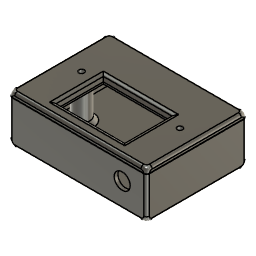
Case (Autodesk Fusion 360 design; units mm, degrees)
part number: 2026-04-11-18-54-48-113
Autodesk Fusion 360 part; units mm, degrees
sketch "Sketch1" plane through (0, 0, 0) normal (0, 0, 1) x (1, 0, 0)
  line L0 (36, -17) -> (-34, -17)
  line L1 (-34, -17) -> (-34, 33)
  line L2 (-34, 33) -> (36, 33)
  line L3 (36, 33) -> (36, -17)
  line L4 (-36, 35) -> (38, 35)
  line L5 (38, 35) -> (38, -19)
  line L6 (38, -19) -> (-36, -19)
  line L7 (-36, -19) -> (-36, 35)
  dimension "d1" = -2
  constraint horizontal L0
  constraint vertical L1
  constraint horizontal L2
  constraint vertical L3
extrude "Extrude1" add sketch "Sketch1" along normal blind 3 contours L0 L1 L2 L3 makes body 1
extrude "Extrude2" add sketch "Sketch1" along normal blind 23 bodies 1
sketch "Sketch2" plane through (-36, 0, 0) normal (-1, 0, 0) x (0, -1, 0)
  line L0 (-35, 0) -> (19, 0)
  line L1 (19, 0) -> (19, 23)
  line L2 (19, 23) -> (-35, 23)
  line L3 (-35, 23) -> (-35, 0)
  line L4 (3.8405, 14.1947) -> (10.2824, 14.1947)
  spline S0 degree 5 poles (10.2824, 14.1947) (10.1277, 14.2067) (9.8414, 14.2278) (9.4814, 14.251) (9.1402, 14.265) (8.9381, 14.255) (8.9359, 14.2207) (9.0834, 14.1681) (9.2938, 14.108) (9.4323, 14.0572) (9.5119, 14.0042) (9.5822, 13.9341) (9.7032, 13.8331) (9.8326, 13.7189) (9.9316, 13.5975) (9.9981, 13.4573) (10.039, 13.2845) (10.0688, 13.0683) (10.0947, 12.8128) (10.114, 12.5387) (10.1198, 12.2727) (10.105, 12.0401) (10.0669, 11.8551) (10.0114, 11.7144) (9.9593, 11.5833) (9.8882, 11.451) (9.7741, 11.3164) (9.6097, 11.1874) (9.4444, 11.0743) (9.3869, 10.985) (9.4842, 10.9238) (9.7088, 10.8991) (9.9628, 10.8944) (10.1702, 10.8974) (10.2835, 10.9005) knots 0 0 0 0 0 0 0.033333 0.066667 0.1 0.133333 0.166667 0.2 0.233333 0.266667 0.3 0.333333 0.366667 0.4 0.433333 0.466667 0.5 0.533333 0.566667 0.6 0.633333 0.666667 0.7 0.733333 0.766667 0.8 0.833333 0.866667 0.9 0.933333 0.966667 1 1 1 1 1 1
  line L5 (10.1343, 12.0688) -> (9.9468, 11.5206)
  line L6 (9.8271, 11.3559) -> (9.3119, 10.9656)
  line L7 (8.9303, 14.2181) -> (9.4188, 14.0666)
  line L8 (9.3851, 14.1073) -> (9.9709, 13.5998)
  line L9 (10.2835, 10.9005) -> (3.8405, 10.9005)
  spline S1 degree 5 poles (10.2824, 14.1947) (10.3107, 14.1924) (10.3649, 14.188) (10.4382, 14.1815) (10.5201, 14.1733) (10.6001, 14.1622) (10.6656, 14.1474) (10.7413, 14.1203) (10.8479, 14.0727) (10.9748, 14.0042) (11.1054, 13.918) (11.221, 13.8196) (11.3211, 13.7164) (11.406, 13.6037) (11.4757, 13.4696) (11.5302, 13.3021) (11.5698, 13.0938) (11.5955, 12.8489) (11.6087, 12.586) (11.6103, 12.3286) (11.6008, 12.1001) (11.5781, 11.9132) (11.5392, 11.7701) (11.4743, 11.6379) (11.3832, 11.4983) (11.2768, 11.3602) (11.1656, 11.2375) (11.0577, 11.1449) (10.9445, 11.0767) (10.8149, 11.0216) (10.6641, 10.9753) (10.5242, 10.9428) (10.4081, 10.9208) (10.3258, 10.9071) (10.2835, 10.9005) knots 0 0 0 0 0 0 0.033333 0.066667 0.1 0.133333 0.166667 0.2 0.233333 0.266667 0.3 0.333333 0.366667 0.4 0.433333 0.466667 0.5 0.533333 0.566667 0.6 0.633333 0.666667 0.7 0.733333 0.766667 0.8 0.833333 0.866667 0.9 0.933333 0.966667 1 1 1 1 1 1
  line L10 (10.4303, 14.2181) -> (10.9188, 14.0666)
  line L11 (10.8851, 14.1073) -> (11.4709, 13.5998)
  line L12 (11.6343, 12.0688) -> (11.4468, 11.5206)
  line L13 (11.3271, 11.3559) -> (10.8119, 10.9656)
  spline S2 degree 5 poles (3.8405, 14.1947) (3.827, 14.1957) (3.7987, 14.1969) (3.7524, 14.1966) (3.6832, 14.1918) (3.585, 14.1778) (3.4774, 14.1546) (3.3667, 14.1181) (3.259, 14.0663) (3.156, 14.0025) (3.0577, 13.9308) (2.9632, 13.854) (2.8723, 13.77) (2.7861, 13.6719) (2.7062, 13.5512) (2.6353, 13.4001) (2.576, 13.2145) (2.5314, 12.9968) (2.5045, 12.7554) (2.4976, 12.5021) (2.5125, 12.2505) (2.5494, 12.0136) (2.6073, 11.8019) (2.683, 11.6212) (2.7715, 11.4716) (2.8677, 11.3495) (2.9685, 11.2496) (3.0732, 11.1659) (3.1882, 11.0945) (3.3197, 11.0332) (3.4705, 10.9806) (3.6079, 10.9447) (3.7205, 10.9213) (3.7998, 10.9072) (3.8405, 10.9005) knots 0 0 0 0 0 0 0.033333 0.066667 0.1 0.133333 0.166667 0.2 0.233333 0.266667 0.3 0.333333 0.366667 0.4 0.433333 0.466667 0.5 0.533333 0.566667 0.6 0.633333 0.666667 0.7 0.733333 0.766667 0.8 0.833333 0.866667 0.9 0.933333 0.966667 1 1 1 1 1 1
  line L14 (3.8606, 14.2596) -> (3.0828, 14.0401)
  line L15 (2.8075, 11.3652) -> (3.311, 10.9966)
  point P0 (9.1746, 14.1424)
  point P1 (9.678, 13.8535)
  point P2 (10.0558, 13.1512)
  point P3 (10.0405, 11.7947)
  point P4 (9.5695, 11.1608)
  point P5 (11.5558, 13.1512)
  point P6 (11.178, 13.8535)
  point P7 (11.5405, 11.7947)
  point P8 (11.0695, 11.1608)
  point P9 (10.6746, 14.1424)
  point P10 (3.4717, 14.1499)
  point P11 (3.011, 13.8917)
  point P12 (2.6182, 13.3365)
  point P13 (2.5919, 11.872)
  point P14 (3.0592, 11.1809)
  constraint horizontal L4
  constraint midpoint P3 L5
  constraint midpoint P4 L6
  constraint midpoint P0 L7
  constraint midpoint P1 L8
  constraint parallel L4 L9
  constraint midpoint P7 L12
  constraint midpoint P8 L13
  constraint midpoint P9 L10
  constraint midpoint P6 L11
  constraint midpoint P10 L14
  constraint midpoint P14 L15
extrude "Extrude3" cut sketch "Sketch2" against normal blind 2 contours L4 S0 L7 L9 S2 bodies 1
sketch "Sketch3" plane through (0, -19, 0) normal (0, -1, 0) x (1, 0, 0)
  line L0 (-36, 0) -> (38, 0)
  line L1 (38, 0) -> (38, 23)
  line L2 (38, 23) -> (-36, 23)
  line L3 (-36, 23) -> (-36, 0)
  circle A0 centre (24.8738, 13.5782) radius 4.325
extrude "Extrude4" cut sketch "Sketch3" against normal blind 2 contours A0 bodies 1
sketch "Sketch4" plane through (0, 0, 23) normal (0, 0, 1) x (-1, 0, 0)
  line L0 (34, -33) -> (-36, -33)
  line L1 (-36, -33) -> (-36, 17)
  line L2 (-36, 17) -> (34, 17)
  line L3 (34, 17) -> (34, -33)
  line L4 (36, 19) -> (-38, 19)
  line L5 (-38, 19) -> (-38, -35)
  line L6 (-38, -35) -> (36, -35)
  line L7 (36, -35) -> (36, 19)
  line L8 (-38, 19) -> (36, 19)
  line L9 (36, 19) -> (36, -35)
  line L10 (36, -35) -> (-38, -35)
  line L11 (-38, -35) -> (-38, 19)
  line L12 (-18.2497, 11.0259) -> (16.2502, 11.0259)
  line L13 (16.2502, 11.0259) -> (16.2502, -11.9741)
  line L14 (16.2502, -11.9741) -> (-18.2497, -11.9741)
  line L15 (-18.2497, -11.9741) -> (-18.2497, 11.0259)
  constraint horizontal L8
  constraint vertical L9
  constraint horizontal L10
  constraint vertical L11
  constraint coincident L6.end L7.start
  constraint coincident L4.end L5.start
  constraint horizontal L12
  constraint vertical L13
  constraint horizontal L14
  constraint vertical L15
extrude "Extrude5" add sketch "Sketch4" along normal blind 3 separate body contours L0 L1 L2 L3 | L4 L5 L6 L7 L8 L9 L10 L11 makes body 2
fillet "Fillet1" radius 1.5 16 edges at (-36, 35, 11.5) (38, 35, 11.5) (-36, -19, 11.5) (1, 35, 0) (-36, 8, 0) (1, -19, 0) (38, -19, 11.5) (38, 8, 0) (-36, 35, 24.5) (38, 35, 24.5) (1, 35, 26) (1, -19, 26) (-36, 8, 26) (38, -19, 24.5) (38, 8, 26) (-36, -19, 24.5) on bodies 1 2
chamfer "Chamfer1" distance 2 angle 45 4 edges at (18.2497, 0.4741, 26) (0.9997, -11.0259, 26) (-16.2502, 0.4741, 26) (0.9997, 11.9741, 26) on bodies 2
fillet "Fillet2" radius 2.5 4 edges at (0.9997, -13.0259, 26) (20.2497, 0.4741, 26) (0.9997, 13.9741, 26) (-18.2502, 0.4741, 26) on bodies 2
sketch "Sketch5" plane through (0, 0, 3) normal (0, 0, 1) x (-1, 0, 0)
  line L0 (-36, -33) -> (34, -33)
  line L1 (34, -33) -> (34, 17)
  line L2 (34, 17) -> (-36, 17)
  line L3 (-36, 17) -> (-36, -33)
  circle A0 centre (-29, -5) radius 4.5
  circle A1 centre (-29, -5) radius 3.5
  dimension "d17" = 9
  dimension "d18" = 7
  constraint concentric A0 A1
  measures "d17" diameter of A0
  measures "d18" diameter of A1
fillet "Fillet3" radius 1 4 edges at (36, -17, 13) (36, 33, 13) (-34, -17, 13) (-34, 33, 13) on bodies 1
sketch "Sketch7" plane through (0, 0, 26) normal (0, 0, 1) x (-1, 0, 0)
  arc A0 (33.0002, -33.5) -> (34.5, -32.0002) centre (33.0002, -32.0002) ccw
  line L0 (34.5, -32.0002) -> (34.5, 16.0002)
  arc A1 (34.5, 16.0002) -> (33.0002, 17.5) centre (33.0002, 16.0002) ccw
  line L1 (33.0002, 17.5) -> (-35.0002, 17.5)
  arc A2 (-35.0002, 17.5) -> (-36.5, 16.0002) centre (-35.0002, 16.0002) ccw
  line L2 (-36.5, 16.0002) -> (-36.5, -32.0002)
  arc A3 (-36.5, -32.0002) -> (-35.0002, -33.5) centre (-35.0002, -32.0002) ccw
  line L3 (-35.0002, -33.5) -> (33.0002, -33.5)
  line L4 (19.2858, 14.0614) -> (19.2858, -15.0096)
  line L5 (19.2858, -15.0096) -> (-21.2852, -15.0096)
  line L6 (-21.2852, -15.0096) -> (-21.2852, 14.0614)
  line L7 (-21.2852, 14.0614) -> (19.2858, 14.0614)
extrude "Extrude10" cut sketch "Sketch2" against normal blind 3 contours L4 S0 L7 | L4 S0 L9 S1 bodies 1
sketch "Sketch8" plane through (0, 0, 3) normal (0, 0, 1) x (-1, 0, 0)
  arc A0 (33, -33) -> (34, -32) centre (33, -32) ccw
  line L0 (34, -32) -> (34, 16)
  arc A1 (34, 16) -> (33, 17) centre (33, 16) ccw
  line L1 (33, 17) -> (-35, 17)
  arc A2 (-35, 17) -> (-36, 16) centre (-35, 16) ccw
  line L2 (-36, 16) -> (-36, -32)
  arc A3 (-36, -32) -> (-35, -33) centre (-35, -32) ccw
  line L3 (-35, -33) -> (33, -33)
  circle A4 centre (25, -9) radius 4.5
  circle A5 centre (-28, -9) radius 4.5
  circle A6 centre (-28, -9) radius 3.5
  circle A7 centre (25, -9) radius 3.5
  dimension "d35" = 9
  dimension "d36" = 9
  dimension "d37" = 7
  dimension "d38" = 7
  constraint concentric A5 A6
  constraint concentric A4 A7
  measures "d35" diameter of A4
  measures "d36" diameter of A5
  measures "d37" diameter of A6
  measures "d38" diameter of A7
extrude "Extrude11" add sketch "Sketch8" along normal blind 20 contours A4 | A5 bodies 1
extrude "Extrude12" cut sketch "Sketch8" against normal blind 2 contours A6 | A7 bodies 1
sketch "Sketch9" plane through (0, 0, 23) normal (0, 0, 1) x (-1, 0, 0)
  circle A0 centre (25, -9) radius 3.5
  circle A1 centre (25, -9) radius 4.5
  circle A2 centre (-28, -9) radius 2.35
  circle A3 centre (25, -9) radius 2.35
  circle A4 centre (-28, -9) radius 3.5
  circle A5 centre (25, -9) radius 3.5
  dimension "d43" = 4.7
  dimension "d44" = 4.7
  dimension "d45" = 7
  constraint concentric A0 A3
  constraint concentric A2 A4
  constraint concentric A3 A5
  measures "d43" diameter of A2
  measures "d44" diameter of A3
  measures "d45" diameter of A4
extrude "Extrude13" add sketch "Sketch9" against normal blind 5 contours A0 A5 | A4 bodies 1
chamfer "Chamfer3" distance 2 angle 45 2 edges at (32.1955, 7.3727, 3) (-20.8045, 7.3727, 3) on bodies 1
sketch "Sketch10" plane through (0, 0, 26) normal (0, 0, 1) x (-1, 0, 0)
  arc A0 (33.0002, -33.5) -> (34.5, -32.0002) centre (33.0002, -32.0002) ccw
  line L0 (34.5, -32.0002) -> (34.5, 16.0002)
  arc A1 (34.5, 16.0002) -> (33.0002, 17.5) centre (33.0002, 16.0002) ccw
  line L1 (33.0002, 17.5) -> (-35.0002, 17.5)
  arc A2 (-35.0002, 17.5) -> (-36.5, 16.0002) centre (-35.0002, 16.0002) ccw
  line L2 (-36.5, 16.0002) -> (-36.5, -32.0002)
  arc A3 (-36.5, -32.0002) -> (-35.0002, -33.5) centre (-35.0002, -32.0002) ccw
  line L3 (-35.0002, -33.5) -> (33.0002, -33.5)
  line L4 (19.2858, 14.0614) -> (19.2858, -15.0096)
  line L5 (19.2858, -15.0096) -> (-21.2852, -15.0096)
  line L6 (-21.2852, -15.0096) -> (-21.2852, 14.0614)
  line L7 (-21.2852, 14.0614) -> (19.2858, 14.0614)
  circle A4 centre (-28, -9) radius 1.45
  circle A5 centre (25, -9) radius 1.45
  dimension "d49" = 2.9
  dimension "d50" = 2.9
  measures "d49" diameter of A4
  measures "d50" diameter of A5
extrude "Extrude14" cut sketch "Sketch10" against normal blind 3 contours A4 | A5 bodies 2
move_body "Move1" bodies 2 to x (1, 0, 0) y (0, 1, 0) z (0, 0, 1) at (-80, 0, -22.5)
move_body "Move2" bodies 2 to x (1, 0, 0) y (0, 1, 0) z (0, 0, 1) at (80, 0, 20)
move_body "Move3" bodies 2 to x (1, 0, 0) y (0, 1, 0) z (0, 0, 1) at (0, 0, 3.1)
move_body "Move4" bodies 2 to x (1, 0, 0) y (0, 1, 0) z (0, 0, 1) at (0, 0, -0.8)
